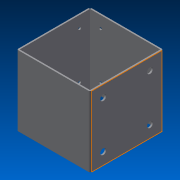
# Autodesk Inventor part: Box
Saved by Autodesk Inventor 2013 (Build 170138000, 138)
## iProperties
Created: 2013-07-15
Part Number: Box
Material: Generic
Document SubType Name: Modeling
Designer: root
Density: 1 g/cm^3
Author: root
Autodesk Inventor part; units mm, degrees
ref_plane "YZ Plane" through (0, 0, 0) normal (1, 0, 0) x (0, 1, 0)
ref_plane "XZ Plane" through (0, 0, 0) normal (0, 1, 0) x (-1, 0, 0)
ref_plane "XY Plane" through (0, 0, 0) normal (0, 0, 1) x (1, 0, 0)
sketch "Sketch4" plane through (0, 0, 0) normal (1, 0, 0) x (0, 1, 0)
  line L0 (0, 0) -> (76.2, 0)
  line L1 (76.2, 0) -> (76.2, 304.8)
  line L2 (76.2, 304.8) -> (0, 304.8)
  line L3 (0, 304.8) -> (0, 0)
  dimension "d7" = 76.2
  dimension "d8" = 304.8
  constraints: 8 end point, 2 parallel, 1 horizontal, 1 perpendicular
  measures "d7" distance of L0.start L0.end
  measures "d8" distance of L2.end L0.start
extrude "Extrusion2" add sketch "Sketch4" along normal blind 1.5875
sketch "Sketch5" plane through (1.5875, 0, 0) normal (1, 0, 0) x (0, 0, -1)
  line L0 (0, 0) -> (0, 76.2) projected
  line L1 (0, 76.2) -> (-304.8, 76.2) projected
  line L2 (-304.8, 76.2) -> (-304.8, 0) projected
  line L3 (-304.8, 0) -> (0, 0) projected
  line L4 (-228.6, 76.2) -> (-228.6, 0)
  line L5 (-152.4, 76.2) -> (-152.4, 0)
  line L6 (-76.2, 76.2) -> (-76.2, 0)
  dimension "d11" = 76.2
  dimension "d12" = 76.2
  dimension "d13" = 76.2
  constraints: 6 end point, 4 point on line, 3 perpendicular, 2 midpoint
  measures "d11" distance between parallel lines of L2 L4
  measures "d12" distance between parallel lines of L0 L6
  measures "d13" distance between parallel lines of L5 L6
bend part "Bend Part2" radius 0.0162 angle 90 line through (1.5875, 76.2, 228.6) along (0, -1, 0) centre toward (1, 0, 0) moving side (0, 0, 1) both sides no
sketch "Sketch6" plane through (1.5875, 0, 0) normal (1, 0, 0) x (0, 0, -1)
  line L0 (-228.6, 0) -> (-228.6, 76.2) projected
  line L1 (-228.6, 0) -> (0, 0) projected
  line L2 (0, 76.2) -> (-228.6, 76.2) projected
  line L3 (-152.4, 76.2) -> (-152.4, 0)
  dimension "d16" = 76.2
  constraints: 2 end point, 2 point on line, 1 perpendicular
  measures "d16" distance between parallel lines of L0 L3
bend part "Bend Part3" radius 0.0162 angle 90 line through (1.5875, 76.2, 152.4) along (0, -1, 0) centre toward (1, 0, 0) moving side (0, 0, 1) both sides no
sketch "Sketch7" plane through (1.5875, 0, 0) normal (1, 0, 0) x (0, 0, -1)
  line L0 (-152.4, 0) -> (-152.4, 76.2) projected
  line L1 (-152.4, 0) -> (0, 0) projected
  line L2 (0, 76.2) -> (-152.4, 76.2) projected
  line L3 (-76.2, 76.2) -> (-76.2, -0.6756)
  dimension "d19" = 76.2
  constraints: 2 end point, 1 midpoint, 1 perpendicular
  measures "d19" distance between parallel lines of L0 L3
bend part "Bend Part4" radius 0.0162 angle 90 line through (1.5875, 76.2, 76.2) along (0, -1, 0) centre toward (1, 0, 0) moving side (0, 0, 1) both sides no
sketch "Sketch8" plane through (77.7783, 0, -1.5783) normal (0, 0, -1) x (-1, 0, 0)
  line L0 (76.1746, 0) -> (0, 0) projected
  line L1 (0, 76.2) -> (76.1746, 76.2) projected
  line L2 (77.7783, 0) -> (77.7783, 76.2) projected
  point P0 (65.0783, 63.5)
  point P1 (65.0783, 12.7)
  dimension "d22" = 12.7
  dimension "d23" = 12.7
  dimension "d24" = 12.7
  dimension "d25" = 12.7
  measures "d22" distance from line of point (65.078, 63.5) L1
  measures "d23" distance from line of L0 point (65.078, 12.7)
  measures "d24" distance from line of point (65.078, 63.5) L2
  measures "d25" distance from line of point (65.078, 12.7) L2
hole "Hole1" at (12.7, 63.5, -1.5783) at (12.7, 12.7, -1.5783) direction (0, 0, 1) diameter 3.175 depth 25.4 tip angle 118
sketch "Sketch9" plane through (0, 0, 0) normal (-1, 0, 0) x (0, 0, 1)
  line L0 (0, 76.2) -> (76.2, 76.2) projected
  line L1 (76.2, 0) -> (0, 0) projected
  line L2 (-1.5783, 76.2) -> (-1.5783, 0) projected
  point P0 (11.1217, 63.5)
  point P1 (11.1217, 12.7)
  dimension "d33" = 12.7
  dimension "d34" = 12.7
  dimension "d35" = 12.7
  dimension "d36" = 12.7
  measures "d33" distance from line of L1 point (11.122, 12.7)
  measures "d34" distance from line of point (11.122, 63.5) L0
  measures "d35" distance from line of L2 point (11.122, 63.5)
  measures "d36" distance from line of L2 point (11.122, 12.7)
hole "Hole2" at (0, 63.5, 11.1217) at (0, 12.7, 11.1217) direction (1, 0, 0) diameter 3.175 depth 25.4 tip angle 118
sketch "Sketch10" plane through (79.3819, 0, 76.2) normal (1, 0, 0) x (0, 0, -1)
  line L0 (0, 76.2) -> (0, 0) projected
  line L1 (76.1746, 0) -> (0, 0) projected
  line L2 (76.1746, 76.2) -> (76.1746, 0) projected
  line L3 (0, 76.2) -> (76.1746, 76.2) projected
  point P0 (76.2, 0)
sketch "Sketch11" plane through (79.3819, 0, 76.2) normal (1, 0, 0) x (0, 0, -1)
  line L0 (76.1746, 76.2) -> (76.1746, 0) projected
  line L1 (0, 76.2) -> (76.1746, 76.2) projected
  line L2 (76.1746, 0) -> (0, 0) projected
  point P0 (76.2, 0)
  point P1 (12.6746, 63.5)
  point P2 (63.4746, 63.5)
  point P3 (12.6746, 12.7)
  point P4 (63.4746, 12.7)
  dimension "d46" = 12.7
  dimension "d47" = 12.7
  dimension "d49" = 12.7
  dimension "d57" = 12.7
  dimension "d58" = 12.7
  dimension "d59" = 50.8
  dimension "d60" = 50.8
  dimension "d61" = 12.7
  measures "d46" distance from line of point (63.475, 63.5) L1
  measures "d47" distance from line of point (12.675, 63.5) L1
  measures "d49" distance from line of point (63.475, 63.5) L0
  measures "d57" distance from line of L2 point (12.675, 12.7)
  measures "d58" distance from line of L2 point (63.475, 12.7)
  measures "d59" distance of point (63.475, 12.7) point (12.675, 12.7)
  measures "d60" distance of point (63.475, 63.5) point (12.675, 63.5)
  measures "d61" distance from line of L0 point (63.475, 12.7)
hole "Hole3" at (79.3819, 63.5, 63.5254) at (79.3819, 63.5, 12.7254) at (79.3819, 12.7, 63.5254) at (79.3819, 12.7, 12.7254) direction (-1, 0, 0) diameter 6.35 depth 25.4 tip angle 118
body "Solid2"
